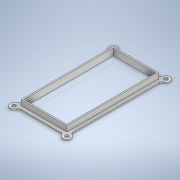
# Autodesk Inventor part: Mount
Saved by Autodesk Inventor 2020.2 (Build 242310000, 310)
## iProperties
Created: 2020-03-28
Part Number: Mount
Material: Generic
Document SubType Name: Modeling
Designer: sdekr
Density: 1 g/cm^3
Appearance: Default
Author: sdekr
## iProperties of the stored document _3DPrint.ipt
Created: 2020-03-28
Part Number: _3DPrint
Material: Generic
Document SubType Name: Modeling
Designer: sdekr
Density: 1 g/cm^3
Appearance: Default
Author: sdekr
Autodesk Inventor part; units mm, degrees
ref_plane "YZ Plane" through (0, 0, 0) normal (1, 0, 0) x (0, 1, 0)
ref_plane "XZ Plane" through (0, 0, 0) normal (0, 1, 0) x (-1, 0, 0)
ref_plane "XY Plane" through (0, 0, 0) normal (0, 0, 1) x (1, 0, 0)
sketch "Sketch1" plane through (0, 0, 0) normal (0, 1, 0) x (-1, 0, 0)
  line L0 (-34.4, 69.4) -> (34.4, 69.4)
  line L1 (34.4, 69.4) -> (34.4, -69.4)
  line L2 (34.4, -69.4) -> (-34.4, -69.4)
  line L3 (-34.4, -69.4) -> (-34.4, 69.4)
  line L4 (-34.4, 69.4) -> (34.4, -69.4) construction
  line L5 (34.4, 69.4) -> (-34.4, -69.4) construction
  line L6 (32.4, -67.4) -> (32.4, 67.4)
  line L7 (32.4, 67.4) -> (-32.4, 67.4)
  line L8 (-32.4, 67.4) -> (-32.4, -67.4)
  line L9 (-32.4, -67.4) -> (32.4, -67.4)
  point P0 (0, 0)
  dimension "d0" = 68.8
  dimension "d1" = 138.8
  dimension "d2" = 2
  constraints: 20 end point, 4 parallel, 2 midpoint, 2 perpendicular, 1 horizontal, 3 other
  measures "d0" distance of L0.start L0.end
  measures "d1" distance of L0.end L1.end
  measures "d2" distance between parallel lines of L1 L6
extrude "Extrusion1" add sketch "Sketch1" along normal blind 10
sketch "Sketch2" plane through (0, 0, 0) normal (0, -1, 0) x (1, 0, 0)
  line L0 (-49.4, 84.4) -> (49.4, 84.4)
  line L1 (49.4, 84.4) -> (49.4, -84.4)
  line L2 (49.4, -84.4) -> (-49.4, -84.4)
  line L3 (-49.4, -84.4) -> (-49.4, 84.4)
  line L4 (-49.4, 84.4) -> (49.4, -84.4) construction
  line L5 (49.4, 84.4) -> (-49.4, -84.4) construction
  line L6 (34.4, 69.4) -> (34.4, -69.4) projected
  line L7 (-34.4, 69.4) -> (34.4, 69.4) projected
  line L8 (34.4, -69.4) -> (-34.4, -69.4) projected
  line L9 (-34.4, -69.4) -> (-34.4, 69.4) projected
  point P0 (0, 0)
  dimension "d5" = 15
  dimension "d6" = 15
  constraints: 12 end point, 2 midpoint, 2 parallel, 1 horizontal, 1 perpendicular
  measures "d5" distance between parallel lines of L1 L6
  measures "d6" distance between parallel lines of L0 L7
extrude "Extrusion2" add sketch "Sketch2" against normal blind 2
fillet "Fillet1" radius 4 4 edges at (49.4, 1, -84.4) (49.4, 1, 84.4) (-49.4, 1, 84.4) (-49.4, 1, -84.4)
sketch "Sketch3" plane through (0, 0, 0) normal (0, -1, 0) x (1, 0, 0)
  arc A0 (-49.4, -80.4) -> (-45.4, -84.4) centre (-45.4, -80.4) ccw projected
  line L0 (-49.4, 80.4) -> (-49.4, -80.4) projected
  arc A1 (-45.4, 84.4) -> (-49.4, 80.4) centre (-45.4, 80.4) ccw projected
  line L1 (45.4, 84.4) -> (-45.4, 84.4) projected
  arc A2 (49.4, 80.4) -> (45.4, 84.4) centre (45.4, 80.4) ccw projected
  line L2 (49.4, -80.4) -> (49.4, 80.4) projected
  arc A3 (45.4, -84.4) -> (49.4, -80.4) centre (45.4, -80.4) ccw projected
  line L3 (-45.4, -84.4) -> (45.4, -84.4) projected
  line L4 (34.4, 69.4) -> (45.4, 80.4)
  circle A4 centre (39.9, 74.9) radius 2.75
  line L5 (34.4, -69.4) -> (-34.4, -69.4) projected
  line L6 (34.4, -69.4) -> (45.4, -80.4)
  circle A5 centre (39.9, -74.9) radius 2.75
  line L7 (45.4, -84.4) -> (-45.4, -84.4) projected
  line L8 (0, -84.4) -> (0, -77.4)
  circle A6 centre (-39.9, 74.9) radius 2.75
  circle A7 centre (-39.9, -74.9) radius 2.75
  point P0 (32.4, -67.4)
  point P1 (32.4, 67.4)
  point P2 (-32.4, 67.4)
  dimension "d20" = 5.5
  dimension "d21" = 5.5
  constraints: 6 end point, 4 centre point, 3 midpoint, 2 symmetric about line, 1 coincident, 1 vertical, 2 other
  measures "d20" diameter of A4
  measures "d21" diameter of A5
extrude "Extrusion3" cut sketch "Sketch3" against normal up to surface (2 mm away) contours A4 L4 | L4 A4 | A5 L6 | L6 A5 | A6 | A7
sketch "Sketch4" plane through (0, 2, 0) normal (0, 1, 0) x (1, 0, 0)
  circle A0 centre (-39.9, -74.9) radius 2.75 projected
  circle A1 centre (-39.9, -74.9) radius 6
  circle A2 centre (39.9, -74.9) radius 2.75 projected
  circle A3 centre (39.9, -74.9) radius 6
  line L0 (33.9209, -74.4) -> (-33.9209, -74.4)
  line L1 (-34.4, -69.4) -> (34.4, -69.4) projected
  line L2 (0, 0) -> (-15.7082, 0)
  circle A4 centre (-39.9, 74.9) radius 2.75
  circle A5 centre (39.9, 74.9) radius 6
  line L3 (33.9209, 74.4) -> (-33.9209, 74.4)
  circle A6 centre (-39.9, 74.9) radius 6
  line L4 (-39.4, -68.9209) -> (-39.4, 68.9209)
  line L5 (-34.4, 69.4) -> (-34.4, -69.4) projected
  line L6 (39.4, -68.9209) -> (39.4, 68.9209)
  line L7 (34.4, -69.4) -> (34.4, 69.4) projected
  circle A7 centre (39.9, 74.9) radius 2.75 projected
  circle A8 centre (-39.9, -74.9) radius 2.75 projected
  circle A9 centre (39.9, -74.9) radius 2.75 projected
  circle A10 centre (-39.9, 74.9) radius 2.75 projected
  arc A11 (-45.4, 84.4) -> (-49.4, 80.4) centre (-45.4, 80.4) ccw projected
  line L8 (-49.4, 80.4) -> (-49.4, -80.4) projected
  arc A12 (-49.4, -80.4) -> (-45.4, -84.4) centre (-45.4, -80.4) ccw projected
  line L9 (-45.4, -84.4) -> (45.4, -84.4) projected
  arc A13 (45.4, -84.4) -> (49.4, -80.4) centre (45.4, -80.4) ccw projected
  line L10 (49.4, -80.4) -> (49.4, 80.4) projected
  arc A14 (49.4, 80.4) -> (45.4, 84.4) centre (45.4, 80.4) ccw projected
  line L11 (45.4, 84.4) -> (-45.4, 84.4) projected
  line L12 (34.4, -69.4) -> (34.4, 69.4) projected
  line L13 (-34.4, -69.4) -> (34.4, -69.4) projected
  line L14 (-34.4, 69.4) -> (-34.4, -69.4) projected
  line L15 (34.4, 69.4) -> (-34.4, 69.4) projected
  dimension "d22" = 12
  dimension "d23" = 12
  dimension "d24" = 5
  dimension "d25" = 5
  dimension "d26" = 5
  constraints: 10 end point, 8 point on circle, 5 centre point, 4 symmetric about line, 3 coincident, 2 horizontal, 2 vertical, 2 other
  measures "d22" diameter of A1
  measures "d23" diameter of A3
  measures "d24" distance between parallel lines of L1 L0
  measures "d25" distance between parallel lines of L4 L5
  measures "d26" distance between parallel lines of L7 L6
extrude "Extrusion4" cut sketch "Sketch4" against normal blind 10 contours L11 A14 L10 A13 L9 A12 L8 A11
fillet "Fillet2" radius 4 8 edges at (-39.4, 1, 68.9209) (-33.9209, 1, 74.4) (-33.9209, 1, -74.4) (-39.4, 1, -68.9209) (33.9209, 1, -74.4) (39.4, 1, -68.9209) (39.4, 1, 68.9209) (33.9209, 1, 74.4)
body "Solid1"
